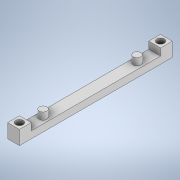
# Autodesk Inventor part: Tamiya-doubleGearBoxStopper
Saved by Autodesk Inventor 2022 (Build 260153000, 153)
## iProperties
Created: 2021-07-11
Part Number: Tamiya-doubleGearBoxStopper
Material: 一般
Document SubType Name: Modeling
Designer: ken
Density: 1 g/cm^3
Appearance: 既定
Author: ken
Autodesk Inventor part; units mm, degrees
ref_plane "YZ Plane" through (0, 0, 0) normal (1, 0, 0) x (0, 1, 0)
ref_plane "XZ Plane" through (0, 0, 0) normal (0, 1, 0) x (-1, 0, 0)
ref_plane "XY Plane" through (0, 0, 0) normal (0, 0, 1) x (1, 0, 0)
sketch "スケッチ1" plane through (0, 0, 0) normal (0, 1, 0) x (-1, 0, 0)
  line L0 (0, 0) -> (5, 0)
  line L1 (5, 0) -> (5, -65)
  line L2 (5, -65) -> (0, -65)
  line L3 (0, -65) -> (0, 0)
  dimension "d0" = 5
  dimension "d1" = 65
  constraints: 8 end point, 2 parallel, 1 horizontal, 1 perpendicular
  measures "d0" distance of L1.end L2.end
  measures "d1" distance of L0.end L1.end
extrude "押し出し1" add sketch "スケッチ1" along normal blind 3
sketch "スケッチ2" plane through (0, 3, 0) normal (0, 1, 0) x (1, 0, 0)
  line L0 (-5, 0) -> (0, 0) projected
  line L1 (-5, 0) -> (0, 0)
  line L2 (0, 0) -> (0, 5)
  line L3 (0, 5) -> (-5, 5)
  line L4 (-5, 5) -> (-5, 0)
  line L5 (0, 65) -> (-5, 65) projected
  line L6 (-5, 65) -> (0, 65)
  line L7 (0, 65) -> (0, 60)
  line L8 (0, 60) -> (-5, 60)
  line L9 (-5, 60) -> (-5, 65)
  dimension "d4" = 5
  dimension "d5" = 5
  dimension "d6" = 5
  dimension "d7" = 5
  constraints: 16 end point, 4 parallel, 2 horizontal, 2 perpendicular
  measures "d4" distance of L3.end L2.end
  measures "d5" distance of L2.end L1.end
  measures "d6" distance of L7.end L8.end
  measures "d7" distance of L6.end L7.end
extrude "押し出し2" add sketch "スケッチ2" along normal blind 3
sketch "スケッチ3" plane through (0, 6, 0) normal (0, 1, 0) x (1, 0, 0)
  line L0 (0, 60) -> (0, 65) projected
  line L1 (0, 65) -> (-5, 65) projected
  line L2 (-5, 0) -> (0, 0) projected
  point P0 (-2.5, 2.5)
  point P1 (-2.5, 62.5)
  dimension "d10" = 2.5
  dimension "d11" = 2.5
  dimension "d12" = 2.5
  constraints: 1 vertical alignment
  measures "d10" distance from line of L0 point (-2.5, 62.5)
  measures "d11" distance from line of L1 point (-2.5, 62.5)
  measures "d12" distance from line of L2 point (-2.5, 2.5)
hole "穴1" at (-2.5, 6, -2.5) at (-2.5, 6, -62.5) direction (0, -1, 0) diameter 3.2 depth 5 tip angle 118
sketch "スケッチ4" plane through (0, 3, 0) normal (0, 1, 0) x (1, 0, 0)
  circle A0 centre (-2.5, 52.5) radius 1.6
  circle A1 centre (-2.5, 12.5) radius 1.6
  line L0 (0, 65) -> (-5, 65) projected
  line L1 (-5, 0) -> (0, 0) projected
  line L2 (-5, 60) -> (-5, 5) projected
  dimension "d20" = 3.2
  dimension "d21" = 3.2
  dimension "d22" = 40
  dimension "d23" = 12.5
  dimension "d24" = 12.5
  dimension "d25" = 2.5
  constraints: 2 centre point, 1 vertical alignment
  measures "d20" diameter of A0
  measures "d21" diameter of A1
  measures "d22" distance of A1.centre A0.centre
  measures "d23" distance from line of L0 A0.centre
  measures "d24" distance from line of L1 A1.centre
  measures "d25" distance from line of L2 A1.centre
extrude "押し出し3" add sketch "スケッチ4" along normal blind 3
